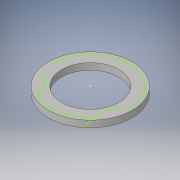
# Autodesk Inventor part: Part1
Saved by Autodesk Inventor 2016 SP1 (Build 200210100, 210)
## iProperties
Created: 2015-11-01
Part Number: Part1
Material: Generic
Document SubType Name: Modeling
Designer: steele
Density: 1 g/cm^3
Appearance: Default
Author: steele
Autodesk Inventor part; units mm, degrees
ref_plane "YZ Plane" through (0, 0, 0) normal (1, 0, 0) x (0, 1, 0)
ref_plane "XZ Plane" through (0, 0, 0) normal (0, 1, 0) x (-1, 0, 0)
ref_plane "XY Plane" through (0, 0, 0) normal (0, 0, 1) x (1, 0, 0)
sketch "Sketch1" plane through (0, 0, 0) normal (0, 1, 0) x (-1, 0, 0)
  point P0 (0, 0)
  point P1 (-56.7479, 47.6171)
  point P2 (-61.2154, 72.9537)
  point P3 (69.6116, 25.3365)
  point P4 (37.0396, 64.1544)
  point P5 (-74.0791, 0)
  point P6 (74.0791, 0)
  constraints: 1 horizontal alignment, 14 other
sketch "Sketch2" plane through (0, 0, 0) normal (0, 1, 0) x (-1, 0, 0)
  circle A0 centre (0, 0) radius 54.991
  circle A1 centre (0, 0) radius 80.391
  dimension "d2" = 109.982
  dimension "d3" = 160.782
  constraints: 2 centre point, 2 coincident
  measures "d2" diameter of A0
  measures "d3" diameter of A1
extrude "Extrusion1" add sketch "Sketch2" against normal blind 12.7
body "Solid1"
